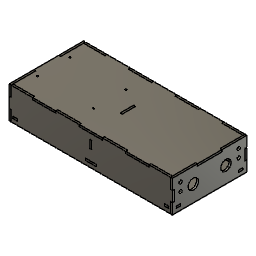
cessna-knobox-enclosure-v77 (Autodesk Fusion 360 design; units mm, degrees)
Autodesk Fusion 360 part; units mm, degrees
sketch "Sketch1" plane through (0, 0, 0) normal (0, 1, 0) x (1, 0, 0)
  line L0 (-146.75, 65) -> (146.75, 65)
  line L1 (146.75, 65) -> (146.75, -65)
  line L2 (146.75, -65) -> (-146.75, -65)
  line L3 (-146.75, -65) -> (-146.75, 65)
  line L4 (-136.75, -30) -> (-33.75, -30) construction
  circle A0 centre (-136.75, -30) radius 1.5
  circle A1 centre (-33.75, -30) radius 1.5
  line L5 (0, 0) -> (0, 38.2702) construction
  line L6 (-150.25, 68.5) -> (150.25, 68.5)
  line L7 (150.25, 68.5) -> (150.25, -68.5)
  line L8 (150.25, -68.5) -> (-150.25, -68.5)
  line L9 (-150.25, -68.5) -> (-150.25, 68.5)
  line L10 (-26.25, -24.7344) -> (-26.25, -4.7344) construction
  line L11 (-136.75, 30) -> (-33.75, 30) construction
  circle A2 centre (-136.75, 30) radius 1.5
  circle A3 centre (-33.75, 30) radius 1.5
  line L12 (-136.75, -30) -> (-136.75, -65) construction
  line L13 (-136.75, 30) -> (-136.75, -30) construction
  line L14 (-136.75, 30) -> (-136.75, 65) construction
  line L15 (0, 0) -> (35, 0) construction
  dimension "d1" = 103
  dimension "d2" = 3
  dimension "d3" = 3
  dimension "d4" = 130
  dimension "d5" = 10
  dimension "d7" = 3.5
  dimension "d9" = 3.5
  dimension "d10" = 3.5
  dimension "d11" = 3.5
  dimension "d20" = 7.5
  dimension "d21" = 173
  dimension "d36" = 103
  dimension "d37" = 3
  dimension "d38" = 3
  dimension "d39" = 60
  constraint horizontal L0
  constraint vertical L1
  constraint horizontal L2
  constraint vertical L3
  constraint horizontal L4
  constraint coincident L4.start A0.centre
  constraint coincident L4.end A1.centre
  constraint coincident L5.start L15.start
  constraint symmetric L0.start L0.end L5
  constraint horizontal L6
  constraint vertical L7
  constraint horizontal L8
  constraint vertical L9
  constraint horizontal L11
  constraint coincident L11.start A2.centre
  constraint coincident L11.end A3.centre
  constraint coincident L2 L12.end
  constraint perpendicular L2 L12
  constraint parallel L12 L13
  constraint coincident L0 L14.end
  constraint perpendicular L0 L14
  constraint equal L12 L14
  constraint perpendicular L5 L15
  constraint symmetric L0.start L2.end L15
  measures "d1" distance of L4.start L4.end
  measures "d2" diameter of A0
  measures "d3" diameter of A1
  measures "d4" distance of L0.start L2.end
  measures "d5" distance of L3 L4.start
  measures "d7" distance of L3 L9
  measures "d9" distance of L0 L6
  measures "d10" distance of L1 L7
  measures "d11" distance of L2 L8
  measures "d20" distance of L4.end L10
  measures "d21" distance of L1 L10
  measures "d36" distance of L11.end L11.start
  measures "d37" diameter of A2
  measures "d38" diameter of A3
  measures "d39" distance of L4 L11
extrude "Extrude1" add sketch "Sketch1" along normal blind 3.5 contours L0 L1 L2 L3 | L6 L7 L8 L9 makes body 1
extrude "Extrude2" add sketch "Sketch1" against normal blind 55 contours L6 L7 L8 L9 bodies 1
sketch "Sketch2" plane through (150.25, 0, 0) normal (1, 0, 0) x (0, 0, -1)
  line L0 (68.5, -55) -> (68.5, 3.5)
  line L1 (68.5, 3.5) -> (-68.5, 3.5)
  line L2 (-68.5, 3.5) -> (-68.5, -55)
  line L3 (-68.5, -55) -> (68.5, -55)
  line L4 (0, 3.5) -> (0, -55) construction
  circle A0 centre (30, -25.025) radius 9.5
  line L5 (68.5, 0) -> (-68.5, 0) construction
  line L6 (30, 0) -> (30, -55) construction
  line L7 (-30, 0) -> (-30, -55) construction
  circle A1 centre (-30, -25.025) radius 9.5
  line L8 (-30, -25.025) -> (30, -25.025) construction
  circle A2 centre (-53.5, -10.025) radius 3
  line L9 (-53.5, 3.5) -> (-53.5, -55) construction
  circle A3 centre (-53.5, -25.025) radius 3
  circle A4 centre (53.5, -10.025) radius 3
  circle A5 centre (53.5, -25.025) radius 3
  line L10 (53.5, 3.5) -> (53.5, -55) construction
  line L11 (-53.5, -10.025) -> (53.5, -10.025) construction
  line L12 (-53.5, -25.025) -> (53.5, -25.025) construction
  point P0 (-30, 0)
  point P1 (30, 0)
  dimension "d16" = 19
  dimension "d17" = 25.025
  dimension "d40" = 19
  dimension "d41" = 6
  dimension "d42" = 15
  dimension "d43" = 6
  dimension "d45" = 6
  dimension "d46" = 6
  dimension "d77" = 15
  constraint midpoint L1 L4.start
  constraint midpoint L3 L4.end
  constraint coincident P1 L6.start
  constraint coincident L3 L6.end
  constraint perpendicular L3 L6
  constraint coincident P0 L7.start
  constraint coincident L3 L7.end
  constraint perpendicular L3 L7
  constraint coincident A0.centre L6
  constraint coincident L7 A1.centre
  constraint coincident A1.centre L8.start
  constraint coincident A0.centre L8.end
  constraint parallel L3 L8
  constraint coincident L1 L9.start
  constraint coincident L3 L9.end
  constraint perpendicular L3 L9
  constraint coincident A2.centre L9
  constraint coincident L9 A3.centre
  constraint coincident L1 L10.start
  constraint coincident L3 L10.end
  constraint perpendicular L3 L10
  constraint symmetric L4 L9.start L10.start
  constraint coincident A4.centre L10
  constraint coincident A5.centre L10
  constraint coincident A2.centre L11.start
  constraint coincident A4.centre L11.end
  constraint coincident A3.centre L12.start
  constraint coincident A5.centre L12.end
  constraint parallel L8 L12
  constraint parallel L8 L11
  constraint coincident A1.centre L12
  measures "d16" diameter of A0
  measures "d17" distance of A0.centre L5
  measures "d40" diameter of A1
  measures "d41" diameter of A2
  measures "d42" distance of L2 L9
  measures "d43" diameter of A3
  measures "d45" diameter of A4
  measures "d46" diameter of A5
  measures "d77" distance of L11 L12
extrude "Extrude3" cut sketch "Sketch2" against normal blind 3.5 contours A0 | A1 | A2 | A3 | A4 | A5 bodies 1
sketch "Sketch3" plane through (0, 0, 68.5) normal (0, 0, 1) x (1, 0, 0)
  line L0 (150.25, -55) -> (150.25, 3.5)
  line L1 (150.25, 3.5) -> (-150.25, 3.5)
  line L2 (-150.25, 3.5) -> (-150.25, -55)
  line L3 (-150.25, -55) -> (150.25, -55)
  line L4 (150.25, 0) -> (-150.25, 0) construction
  line L5 (-150.25, -51.5) -> (150.25, -51.5) construction
  line L6 (-146.75, 3.5) -> (-146.75, -55) construction
  line L7 (146.75, 3.5) -> (146.75, -55) construction
  line L8 (0, 3.5) -> (0, -55) construction
  line L9 (-107.3214, 3.5) -> (-107.3214, -55) construction
  line L10 (-64.3929, 3.5) -> (-64.3929, -55) construction
  line L11 (-21.4643, 3.5) -> (-21.4643, -55) construction
  line L12 (21.4643, 3.5) -> (21.4643, -55) construction
  line L13 (64.3929, 3.5) -> (64.3929, -55) construction
  line L14 (107.3214, 3.5) -> (107.3214, -55) construction
  line L15 (-150.25, -25.75) -> (-107.3214, -25.75) construction
  line L16 (-107.3214, -25.75) -> (-64.3929, -25.75) construction
  line L17 (-64.3929, -25.75) -> (-21.4643, -25.75) construction
  line L18 (-21.4643, -25.75) -> (21.4643, -25.75) construction
  line L19 (21.4643, -25.75) -> (64.3929, -25.75) construction
  line L20 (64.3929, -25.75) -> (107.3214, -25.75) construction
  line L21 (107.3214, -25.75) -> (150.25, -25.75) construction
  line L22 (-150.25, -16) -> (150.25, -16) construction
  line L23 (-150.25, -35.5) -> (150.25, -35.5) construction
  line L24 (-127.3214, 3.5) -> (-127.3214, -16) construction
  line L25 (-127.3214, -16) -> (-127.3214, -35.5) construction
  line L26 (-127.3214, -35.5) -> (-127.3214, -55) construction
  line L27 (-150.25, -16) -> (-146.75, -16)
  line L28 (-146.75, -16) -> (-146.75, 3.5)
  line L29 (-107.3214, 3.5) -> (-107.3214, 0)
  line L30 (-107.3214, 0) -> (-64.3929, 0)
  line L31 (-64.3929, 0) -> (-64.3929, 3.5)
  line L32 (-21.4643, 3.5) -> (-21.4643, 0)
  line L33 (-21.4643, 0) -> (21.4643, 0)
  line L34 (21.4643, 0) -> (21.4643, 3.5)
  line L35 (64.3929, 3.5) -> (64.3929, 0)
  line L36 (64.3929, 0) -> (107.3214, 0)
  line L37 (107.3214, 0) -> (107.3214, 3.5)
  line L38 (146.75, 3.5) -> (146.75, -16)
  line L39 (146.75, -16) -> (150.25, -16)
  line L40 (-150.25, -35.5) -> (-146.75, -35.5)
  line L41 (-146.75, -35.5) -> (-146.75, -55)
  line L42 (150.25, -35.5) -> (146.75, -35.5)
  line L43 (146.75, -35.5) -> (146.75, -55)
  dimension "d22" = 3.5
  dimension "d23" = 3.5
  dimension "d24" = 3.5
  dimension "d25" = 20
  constraint coincident L2 L5.start
  constraint coincident L0 L5.end
  constraint perpendicular L0 L5
  constraint coincident L1 L6.start
  constraint coincident L3 L6.end
  constraint perpendicular L3 L6
  constraint coincident L1 L7.start
  constraint coincident L3 L7.end
  constraint perpendicular L3 L7
  constraint midpoint L1 L8.start
  constraint midpoint L3 L8.end
  constraint coincident L1 L9.start
  constraint coincident L3 L9.end
  constraint perpendicular L3 L9
  constraint coincident L1 L10.start
  constraint coincident L3 L10.end
  constraint perpendicular L5 L10
  constraint coincident L1 L11.start
  constraint coincident L3 L11.end
  constraint perpendicular L3 L11
  constraint coincident L1 L12.start
  constraint coincident L3 L12.end
  constraint perpendicular L3 L12
  constraint coincident L1 L13.start
  constraint coincident L3 L13.end
  constraint perpendicular L3 L13
  constraint coincident L1 L14.start
  constraint coincident L3 L14.end
  constraint perpendicular L3 L14
  constraint midpoint L2 L15.start
  constraint midpoint L9 L15.end
  constraint midpoint L10 L16.end
  constraint midpoint L11 L17.end
  constraint midpoint L12 L18.end
  constraint midpoint L13 L19.end
  constraint midpoint L14 L20.end
  constraint midpoint L0 L21.end
  constraint equal L15 L16
  constraint equal L16 L17
  constraint equal L17 L18
  constraint equal L18 L19
  constraint equal L19 L20
  constraint equal L20 L21
  constraint coincident L2 L22.start
  constraint coincident L0 L22.end
  constraint perpendicular L0 L22
  constraint coincident L2 L23.start
  constraint coincident L0 L23.end
  constraint perpendicular L0 L23
  constraint coincident L1 L24.start
  constraint coincident L22 L24.end
  constraint perpendicular L22 L24
  constraint coincident L23 L25.end
  constraint perpendicular L23 L25
  constraint coincident L3 L26.end
  constraint perpendicular L3 L26
  constraint equal L25 L26
  constraint equal L24 L25
  constraint coincident L6 L27.end
  constraint coincident L22 L27.end
  constraint coincident L4 L29.end
  constraint coincident L9 L29.end
  constraint coincident L4 L30.end
  constraint coincident L10 L30.end
  constraint coincident L4 L32.end
  constraint coincident L11 L32.end
  constraint coincident L4 L33.end
  constraint coincident L12 L33.end
  constraint coincident L4 L35.end
  constraint coincident L13 L35.end
  constraint coincident L4 L36.end
  constraint coincident L14 L36.end
  constraint coincident L7 L38.end
  constraint coincident L22 L38.end
  constraint coincident L6 L40.end
  constraint coincident L23 L40.end
  constraint coincident L7 L42.end
  constraint coincident L23 L42.end
  measures "d22" distance of L3 L5
  measures "d23" distance of L2 L6
  measures "d24" distance of L0 L7
  measures "d25" distance of L9 L24
sketch "Sketch4" plane through (0, 0, -68.5) normal (0, 0, -1) x (-1, 0, 0)
  line L0 (150.25, -55) -> (150.25, 3.5)
  line L1 (150.25, 3.5) -> (-150.25, 3.5)
  line L2 (-150.25, 3.5) -> (-150.25, -55)
  line L3 (-150.25, -55) -> (150.25, -55)
  line L4 (146.75, 3.5) -> (146.75, -55) construction
  line L5 (107.3214, 3.5) -> (107.3214, -55) construction
  line L6 (64.3929, 3.5) -> (64.3929, -55) construction
  line L7 (21.4643, 3.5) -> (21.4643, -55) construction
  line L8 (-21.4643, 3.5) -> (-21.4643, -55) construction
  line L9 (-64.3929, 3.5) -> (-64.3929, -55) construction
  line L10 (-107.3214, 3.5) -> (-107.3214, -55) construction
  line L11 (150.25, -16) -> (-150.25, -16) construction
  line L12 (150.25, -35.5) -> (-150.25, -35.5) construction
  line L13 (-146.75, 3.5) -> (-146.75, -55) construction
  line L14 (-150.25, -16) -> (-146.75, -16)
  line L15 (-146.75, -16) -> (-146.75, 3.5)
  line L16 (-150.25, 0) -> (150.25, 0) construction
  line L17 (-107.3214, 3.5) -> (-107.3214, 0)
  line L18 (-107.3214, 0) -> (-64.3929, 0)
  line L19 (-64.3929, 0) -> (-64.3929, 3.5)
  line L20 (-21.4643, 3.5) -> (-21.4643, 0)
  line L21 (-21.4643, 0) -> (21.4643, 0)
  line L22 (21.4643, 0) -> (21.4643, 3.5)
  line L23 (64.3929, 3.5) -> (64.3929, 0)
  line L24 (64.3929, 0) -> (107.3214, 0)
  line L25 (107.3214, 0) -> (107.3214, 3.5)
  line L26 (146.75, 3.5) -> (146.75, -16)
  line L27 (146.75, -16) -> (150.25, -16)
  line L28 (150.25, -35.5) -> (146.75, -35.5)
  line L29 (146.75, -35.5) -> (146.75, -55)
  line L30 (-150.25, -35.5) -> (-146.75, -35.5)
  line L31 (-146.75, -35.5) -> (-146.75, -55)
  constraint coincident L11.end L14.start
  constraint coincident L13 L14.end
  constraint coincident L11 L14.end
  constraint coincident L13.start L15.end
  constraint coincident L10.start L17.start
  constraint coincident L10 L17.end
  constraint coincident L16 L17.end
  constraint coincident L9 L18.end
  constraint coincident L16 L18.end
  constraint coincident L9.start L19.end
  constraint coincident L8.start L20.start
  constraint coincident L8 L20.end
  constraint coincident L16 L20.end
  constraint coincident L7 L21.end
  constraint coincident L16 L21.end
  constraint coincident L7.start L22.end
  constraint coincident L6.start L23.start
  constraint coincident L6 L23.end
  constraint coincident L16 L23.end
  constraint coincident L5 L24.end
  constraint coincident L16 L24.end
  constraint coincident L5.start L25.end
  constraint coincident L4.start L26.start
  constraint coincident L4 L26.end
  constraint coincident L11 L26.end
  constraint coincident L11.start L27.end
  constraint coincident L12.start L28.start
  constraint coincident L4 L28.end
  constraint coincident L12 L28.end
  constraint coincident L4.end L29.end
  constraint coincident L12.end L30.start
  constraint coincident L12 L30.end
  constraint coincident L13 L30.end
  constraint coincident L13.end L31.end
extrude "Extrude4" add sketch "Sketch3" against normal blind 3.5 separate body contours L0 L1 L2 L3 L27 L28 L29 L30 L31 L32 L33 L34 L35 L36 L37 L38 L39 L40 L41 L42 L43 makes body 2
extrude "Extrude5" add sketch "Sketch4" against normal blind 3.5 separate body contours L0 L1 L2 L3 L14 L15 L17 L18 L19 L20 L21 L22 L23 L24 L25 L26 L27 L28 L29 L30 L31 makes body 3
combine "Combine1" operation cut target body 1 tool bodies 2 3 keep tools
sketch "Sketch5" plane through (150.25, 0, 0) normal (1, 0, 0) x (0, 0, -1)
  circle A0 centre (30, -25.025) radius 9.5
  line L0 (68.5, -35.5) -> (65, -35.5)
  line L1 (65, -35.5) -> (65, -16)
  line L2 (65, -16) -> (68.5, -16)
  line L3 (68.5, -16) -> (68.5, 3.5)
  line L4 (68.5, 3.5) -> (-68.5, 3.5)
  line L5 (-68.5, 3.5) -> (-68.5, -16)
  line L6 (-68.5, -16) -> (-65, -16)
  line L7 (-65, -16) -> (-65, -35.5)
  line L8 (-65, -35.5) -> (-68.5, -35.5)
  line L9 (-68.5, -35.5) -> (-68.5, -55)
  line L10 (-68.5, -55) -> (68.5, -55)
  line L11 (68.5, -55) -> (68.5, -35.5)
  line L12 (0, 3.5) -> (0, -55) construction
  line L13 (-22.8333, 3.5) -> (-22.8333, -55) construction
  line L14 (22.8333, 3.5) -> (22.8333, -55) construction
  line L15 (-68.5, -45.25) -> (-22.8333, -45.25) construction
  line L16 (-22.8333, -45.25) -> (22.8333, -45.25) construction
  line L17 (22.8333, -45.25) -> (68.5, -45.25) construction
  line L18 (-68.5, 0) -> (68.5, 0) construction
  line L19 (-22.8333, 3.5) -> (-22.8333, 0)
  line L20 (-22.8333, 0) -> (22.8333, 0)
  line L21 (22.8333, 0) -> (22.8333, 3.5)
  circle A1 centre (-30, -25.025) radius 9.5
  circle A2 centre (-53.5, -25.025) radius 3
  circle A3 centre (53.5, -10.025) radius 3
  circle A4 centre (-53.5, -10.025) radius 3
  circle A5 centre (53.5, -25.025) radius 3
  dimension "d31" = 3.5
  constraint midpoint L4 L12.start
  constraint midpoint L10 L12.end
  constraint coincident L4 L13.start
  constraint coincident L10 L13.end
  constraint perpendicular L10 L13
  constraint coincident L4 L14.start
  constraint coincident L10 L14.end
  constraint perpendicular L10 L14
  constraint symmetric L12 L13 L14
  constraint midpoint L9 L15.start
  constraint coincident L13 L15.end
  constraint perpendicular L13 L15
  constraint coincident L14 L16.end
  constraint perpendicular L14 L16
  constraint midpoint L11 L17.end
  constraint perpendicular L11 L17
  constraint equal L16 L17
  constraint coincident L5 L18.start
  constraint coincident L3 L18.end
  constraint perpendicular L3 L18
  constraint coincident L18 L19.end
  constraint coincident L13 L19.end
  constraint coincident L18 L20.end
  constraint coincident L14 L20.end
  measures "d31" distance of L4 L18
extrude "Extrude6" add sketch "Sketch5" against normal blind 3.5 separate body contours L0 L1 L2 L3 L4 L5 L6 L7 L8 L9 L10 L11 L19 L20 L21 makes body 4
sketch "Sketch6" plane through (-150.25, 0, 0) normal (-1, 0, 0) x (0, 0, 1)
  line L0 (-68.5, -16) -> (-65, -16)
  line L1 (-65, -16) -> (-65, -35.5)
  line L2 (-65, -35.5) -> (-68.5, -35.5)
  line L3 (-68.5, -35.5) -> (-68.5, -55)
  line L4 (-68.5, -55) -> (68.5, -55)
  line L5 (68.5, -55) -> (68.5, -35.5)
  line L6 (68.5, -35.5) -> (65, -35.5)
  line L7 (65, -35.5) -> (65, -16)
  line L8 (65, -16) -> (68.5, -16)
  line L9 (68.5, -16) -> (68.5, 3.5)
  line L10 (68.5, 3.5) -> (-68.5, 3.5)
  line L11 (-68.5, 3.5) -> (-68.5, -16)
  line L12 (-22.8333, 0) -> (-22.8333, 3.5)
  line L13 (22.8333, 0) -> (-22.8333, 0)
  line L14 (22.8333, 3.5) -> (22.8333, 0)
extrude "Extrude7" add sketch "Sketch6" against normal blind 3.5 separate body contours L0 L1 L2 L3 L4 L5 L6 L7 L8 L9 L10 L11 L12 L13 L14 makes body 5
combine "Combine2" operation cut target body 1 tool bodies 4 5 keep tools
sketch "Sketch7" plane through (-150.25, 0, 0) normal (-1, 0, 0) x (0, 0, 1)
  line L0 (22.8333, 3.5) -> (22.8333, 0)
  line L1 (22.8333, 0) -> (-22.8333, 0)
  line L2 (-22.8333, 0) -> (-22.8333, 3.5)
  line L3 (-22.8333, 3.5) -> (-68.5, 3.5)
  line L4 (-68.5, 3.5) -> (-68.5, -16)
  line L5 (-68.5, -16) -> (-65, -16)
  line L6 (-65, -16) -> (-65, -35.5)
  line L7 (-65, -35.5) -> (-68.5, -35.5)
  line L8 (-68.5, -35.5) -> (-68.5, -55)
  line L9 (-68.5, -55) -> (68.5, -55)
  line L10 (68.5, -55) -> (68.5, -35.5)
  line L11 (68.5, -35.5) -> (65, -35.5)
  line L12 (65, -35.5) -> (65, -16)
  line L13 (65, -16) -> (68.5, -16)
  line L14 (68.5, -16) -> (68.5, 3.5)
  line L15 (68.5, 3.5) -> (22.8333, 3.5)
sketch "Sketch12" plane through (-150.25, -23.25, 0) normal (-1, 0, 0) x (0, 0, 1)
  line L0 (0, 23.25) -> (0, -25) construction
  circle A0 centre (-15, 8.25) radius 1.5
  circle A1 centre (15, 8.25) radius 1.5
  line L1 (-15, 8.25) -> (15, 8.25) construction
  line L2 (68.5, 23.25) -> (-68.5, 23.25) construction
  circle A2 centre (-30, -1.775) radius 9.5 construction
  circle A3 centre (30, -1.775) radius 9.5 construction
  line L3 (-30, -1.775) -> (-30, -27) construction
  line L4 (-68.5, -31.75) -> (68.5, -31.75) construction
  line L5 (-6.02, 13.7) -> (6.02, 13.7)
  line L6 (6.02, 13.7) -> (6.02, 2.8)
  line L7 (6.02, 2.8) -> (-6.02, 2.8)
  line L8 (-6.02, 2.8) -> (-6.02, 13.7)
  point P0 (0, 23.25)
  dimension "d47" = 3
  dimension "d48" = 3
  dimension "d49" = 30
  dimension "d52" = 10.9
  dimension "d53" = 12.04
  dimension "d56" = 15
  constraint coincident P0 L0.start
  constraint vertical L0
  constraint coincident A0.centre L1.start
  constraint coincident A1.centre L1.end
  constraint perpendicular L0 L1
  constraint symmetric L0 A0.centre A1.centre
  constraint coincident A2.centre L3.start
  constraint perpendicular L1 L3
  constraint horizontal L5
  constraint vertical L6
  constraint horizontal L7
  constraint vertical L8
  constraint symmetric L0 L6.end L7.end
  constraint symmetric L1 L5.start L7.end
  measures "d47" diameter of A0
  measures "d48" diameter of A1
  measures "d49" distance of A0.centre A1.centre
  measures "d52" distance of L5.start L7.end
  measures "d53" distance of L5.start L5.end
  measures "d56" distance of L1 L2
extrude "Extrude8" cut sketch "Sketch12" against normal blind 3.5 bodies 5
ref_plane "WorkPlane1" through (-148.5, -51.5, 0) normal (0, -1, 0) x (0, 0, -1)
sketch "Sketch13" plane through (-148.5, -51.5, 0) normal (0, -1, 0) x (1, 0, 0)
  line L0 (1.75, 68.5) -> (1.75, -68.5)
  line L1 (1.75, -65) -> (295.25, -65)
  line L2 (1.75, -65) -> (1.75, -50)
  arc A0 (16.75, -65) -> (1.75, -50) centre (1.75, -65) ccw
  line L3 (1.75, -65) -> (16.75, -65)
  dimension "d58" = 15
  constraint coincident L1.start L2.start
  constraint perpendicular L1 L2
  measures "d58" distance of L1.start L2.end
extrude "Extrude9" add sketch "Sketch13" against normal blind 10.5 separate body makes body 6
ref_plane "WorkPlane2" through (-139.25, -48, -57.5) normal (0, -1, 0) x (1, 0, 0)
ref_plane "WorkPlane3" through (-139.25, -44.5, -57.5) normal (0, -1, 0) x (1, 0, 0)
split "Split1" by plane through (-139.25, -44.5, -57.5) normal (0, -1, 0) and through (-139.25, -48, -57.5) normal (0, -1, 0) bodies 6 makes body 7 at (-143.9112, -45.6667, -50.2711) makes body 8 at (-144.6298, -51.5, -55.2534)
sketch "Sketch14" plane through (0, 0, -65) normal (0, 0, -1) x (-1, 0, 0)
  line L0 (131.75, -48) -> (146.75, -48)
  line L1 (146.75, -48) -> (146.75, -44.5)
  line L2 (146.75, -44.5) -> (131.75, -44.5)
  line L3 (131.75, -44.5) -> (131.75, -48)
  line L4 (139.25, -44.5) -> (139.25, -48) construction
  line L5 (135.25, -44.5) -> (135.25, -48)
  line L6 (143.25, -44.5) -> (143.25, -48)
  dimension "d63" = 8
  constraint midpoint L2 L4.start
  constraint midpoint L0 L4.end
  constraint coincident L2 L5.start
  constraint coincident L0 L5.end
  constraint perpendicular L0 L5
  constraint coincident L2 L6.start
  constraint coincident L0 L6.end
  constraint perpendicular L0 L6
  constraint symmetric L4 L5.start L6.start
  measures "d63" distance of L5 L6
extrude "Extrude10" add sketch "Sketch14" along normal blind 3.5 contours L0 L2 L5 L6 bodies 7
sketch "Sketch15" plane through (-146.75, 0, 0) normal (-1, 0, 0) x (0, 0, 1)
  line L0 (-65, -48) -> (-50, -48)
  line L1 (-50, -48) -> (-50, -44.5)
  line L2 (-50, -44.5) -> (-65, -44.5)
  line L3 (-65, -44.5) -> (-65, -48)
  line L4 (-57.5, -44.5) -> (-57.5, -48) construction
  line L5 (-61.5, -44.5) -> (-61.5, -48)
  line L6 (-53.5, -44.5) -> (-53.5, -48)
  dimension "d66" = 8
  constraint midpoint L2 L4.start
  constraint midpoint L0 L4.end
  constraint coincident L2 L5.start
  constraint coincident L0 L5.end
  constraint perpendicular L0 L5
  constraint coincident L2 L6.start
  constraint coincident L0 L6.end
  constraint perpendicular L0 L6
  constraint symmetric L4 L5.start L6.start
  measures "d66" distance of L5 L6
extrude "Extrude11" add sketch "Sketch15" along normal blind 3.5 contours L0 L2 L5 L6 bodies 7
sketch "Sketch16" plane through (0, -48, 0) normal (0, -1, 0) x (1, 0, 0)
  line L0 (-146.75, -65) -> (-143.25, -65)
  line L1 (-143.25, -65) -> (-143.25, -68.5)
  line L2 (-143.25, -68.5) -> (-135.25, -68.5)
  line L3 (-135.25, -68.5) -> (-135.25, -65)
  line L4 (-135.25, -65) -> (-131.75, -65)
  arc A0 (-131.75, -65) -> (-146.75, -50) centre (-146.75, -65) ccw
  line L5 (-146.75, -50) -> (-146.75, -53.5)
  line L6 (-146.75, -53.5) -> (-150.25, -53.5)
  line L7 (-150.25, -53.5) -> (-150.25, -61.5)
  line L8 (-150.25, -61.5) -> (-146.75, -61.5)
  line L9 (-146.75, -61.5) -> (-146.75, -65)
  line L10 (-142.5, -55.9689) -> (-144.25, -59)
  line L11 (-144.25, -59) -> (-142.5, -62.0311)
  line L12 (-142.5, -62.0311) -> (-139, -62.0311)
  line L13 (-139, -62.0311) -> (-137.25, -59)
  line L14 (-137.25, -59) -> (-139, -55.9689)
  line L15 (-139, -55.9689) -> (-142.5, -55.9689)
  line L16 (-150.25, -59) -> (-133.0023, -59) construction
  line L17 (-140.75, -68.5) -> (-140.75, -51.2523) construction
  point P0 (-140.75, -59)
  dimension "d69" = 3.5
  dimension "d70" = 2.5
  dimension "d71" = 2.5
  constraint coincident L7 L16.start
  constraint coincident A0 L16.end
  constraint perpendicular L7 L16
  constraint coincident L2 L17.start
  constraint coincident A0 L17.end
  constraint perpendicular L16 L17
  constraint coincident P0 L16
  constraint coincident P0 L17
  constraint parallel L15 L16
  measures "d69" distance of L10.start P0
  measures "d70" distance of L8 L16
  measures "d71" distance of L1 L17
extrude "Extrude12" cut sketch "Sketch16" against normal blind 3.5 contours L10 L11 L12 L13 L14 L15 bodies 7
sketch "Sketch17" plane through (0, -51.5, 0) normal (0, -1, 0) x (1, 0, 0)
  line L0 (-146.75, -65) -> (-131.75, -65)
  arc A0 (-131.75, -65) -> (-146.75, -50) centre (-146.75, -65) ccw
  line L1 (-146.75, -50) -> (-146.75, -65)
  line L2 (-139, -55.9689) -> (-142.5, -55.9689) construction
  line L3 (-142.5, -55.9689) -> (-144.25, -59) construction
  line L4 (-144.25, -59) -> (-142.5, -62.0311) construction
  line L5 (-142.5, -62.0311) -> (-139, -62.0311) construction
  line L6 (-139, -62.0311) -> (-137.25, -59) construction
  line L7 (-137.25, -59) -> (-139, -55.9689) construction
  circle A1 centre (-140.75, -59) radius 1.5
  point P0 (-140.75, -59)
  dimension "d74" = 3
  constraint coincident P0 A1.centre
  measures "d74" diameter of A1
extrude "Extrude13" cut sketch "Sketch17" against normal blind 10.5 contours A1 bodies 6 8
copy_body "CopyPasteBodies1" bodies 7 8 6 makes body 9 makes body 10 makes body 11
move_body "Move1" bodies 9 10 11 to x (0, 0, 1) y (0, 1, 0) z (-1, 0, 0) at (81.75, 0, 81.75)
copy_body "CopyPasteBodies2" bodies 9 10 11 makes body 12 makes body 13 makes body 14
move_body "Move2" bodies 12 13 14 to x (0, 0, 1) y (0, 1, 0) z (-1, 0, 0) at (81.75, 0, -81.75)
copy_body "CopyPasteBodies3" bodies 6 7 8 makes body 15 makes body 16 makes body 17
move_body "Move3" bodies 15 16 17 to x (0, 0, -1) y (0, 1, 0) z (1, 0, 0) at (-81.75, 0, -81.75)
combine "Combine3" operation cut target body 2 tool bodies 16 12 keep tools
combine "Combine4" operation cut target body 3 tool bodies 7 9 keep tools
combine "Combine5" operation cut target body 5 tool bodies 16 7 keep tools
combine "Combine6" operation cut target body 4 tool bodies 12 9 keep tools
ref_plane "WorkPlane4" through (-1.75, -25.75, 0) normal (1, 0, 0) x (0, 0, -1)
sketch "Sketch19" plane through (-1.75, -25.75, 0) normal (1, 0, 0) x (0, 0, -1)
  line L0 (-65, 9.75) -> (-65, -9.75)
  line L1 (65, -9.75) -> (65, 9.75)
  line L2 (-22.8333, 25.75) -> (22.8333, 25.75)
  line L3 (-65, -9.75) -> (-65, 25.75)
  line L4 (-65, 25.75) -> (65, 25.75)
  line L5 (65, 25.75) -> (65, -9.75)
  line L6 (-65, -9.75) -> (-61, -9.75)
  line L7 (-61, -9.75) -> (-61, 21.75)
  line L8 (-61, 21.75) -> (61, 21.75)
  line L9 (65, -9.75) -> (61, -9.75)
  line L10 (61, -9.75) -> (61, 21.75)
  dimension "d81" = 4
  dimension "d82" = 4
  dimension "d83" = 4
  constraint coincident L0.end L3.start
  constraint perpendicular L2 L3
  constraint perpendicular L1 L4
  constraint coincident L1.start L5.end
  constraint perpendicular L4 L5
  constraint coincident L2.end L4
  constraint perpendicular L3 L6
  constraint perpendicular L4 L7
  constraint perpendicular L5 L8
  constraint perpendicular L1 L9
  constraint perpendicular L4 L10
  measures "d81" distance of L0.end L6.end
  measures "d82" distance of L4 L8
  measures "d83" distance of L1.start L9.end
extrude "Extrude16" add sketch "Sketch19" along normal blind 3.5 separate body makes body 18
sketch "Sketch20" plane through (0, 0, -65) normal (0, 0, -1) x (-1, 0, 0)
  line L0 (1.75, -35.5) -> (1.75, 0)
  line L1 (1.75, 0) -> (-1.75, 0)
  line L2 (-1.75, 0) -> (-1.75, -35.5)
  line L3 (-1.75, -35.5) -> (1.75, -35.5)
  line L4 (-1.75, -17.75) -> (1.75, -17.75) construction
  line L5 (-1.75, -10.25) -> (1.75, -10.25)
  line L6 (-1.75, -25.25) -> (1.75, -25.25)
  dimension "d88" = 15
  constraint midpoint L2 L4.start
  constraint midpoint L0 L4.end
  constraint coincident L2 L5.start
  constraint coincident L0 L5.end
  constraint perpendicular L0 L5
  constraint coincident L2 L6.start
  constraint coincident L0 L6.end
  constraint perpendicular L0 L6
  constraint symmetric L4 L5.start L6.start
  measures "d88" distance of L5 L6
extrude "Extrude17" add sketch "Sketch20" along normal blind 3.5 contours L0 L2 L5 L6 bodies 18
sketch "Sketch21" plane through (0, 0, 65) normal (0, 0, 1) x (1, 0, 0)
  line L0 (-1.75, 0) -> (-1.75, -35.5)
  line L1 (-1.75, -35.5) -> (1.75, -35.5)
  line L2 (1.75, -35.5) -> (1.75, 0)
  line L3 (1.75, 0) -> (-1.75, 0)
  line L4 (1.75, -10.25) -> (-1.75, -10.25)
  line L5 (1.75, -25.25) -> (-1.75, -25.25)
extrude "Extrude18" add sketch "Sketch21" along normal blind 3.5 contours L0 L2 L4 L5 bodies 18
sketch "Sketch22" plane through (0, 0, 0) normal (0, 1, 0) x (-1, 0, 0)
  line L0 (1.75, -65) -> (1.75, 65)
  line L1 (1.75, 65) -> (-1.75, 65)
  line L2 (-1.75, 65) -> (-1.75, -65)
  line L3 (-1.75, -65) -> (1.75, -65)
  line L4 (1.75, 0) -> (-1.75, 0) construction
  line L5 (1.75, -12.5) -> (-1.75, -12.5)
  line L6 (1.75, 12.5) -> (-1.75, 12.5)
  dimension "d93" = 25
  constraint midpoint L0 L4.start
  constraint midpoint L2 L4.end
  constraint coincident L0 L5.start
  constraint coincident L2 L5.end
  constraint perpendicular L2 L5
  constraint coincident L0 L6.start
  constraint coincident L2 L6.end
  constraint perpendicular L2 L6
  constraint symmetric L4 L5.end L6.end
  measures "d93" distance of L5 L6
extrude "Extrude19" add sketch "Sketch22" along normal blind 3.5 contours L0 L2 L5 L6 bodies 18
combine "Combine7" operation cut target body 1 tool bodies 18 keep tools
combine "Combine8" operation cut target body 2 tool bodies 18 keep tools
combine "Combine9" operation cut target body 3 tool bodies 18 keep tools
sketch "bottom" plane through (0, 3.5, 0) normal (0, 1, 0) x (-1, 0, 0)
  line L0 (-1.75, 12.5) -> (1.75, 12.5)
  line L1 (1.75, 12.5) -> (1.75, -12.5)
  line L2 (1.75, -12.5) -> (-1.75, -12.5)
  line L3 (-1.75, -12.5) -> (-1.75, 12.5)
  line L4 (146.75, -22.8333) -> (150.25, -22.8333)
  line L5 (150.25, -22.8333) -> (150.25, 22.8333)
  line L6 (150.25, 22.8333) -> (146.75, 22.8333)
  line L7 (146.75, 22.8333) -> (146.75, 65)
  line L8 (146.75, 65) -> (107.3214, 65)
  line L9 (107.3214, 65) -> (107.3214, 68.5)
  line L10 (107.3214, 68.5) -> (64.3929, 68.5)
  line L11 (64.3929, 68.5) -> (64.3929, 65)
  line L12 (64.3929, 65) -> (21.4643, 65)
  line L13 (21.4643, 65) -> (21.4643, 68.5)
  line L14 (21.4643, 68.5) -> (-21.4643, 68.5)
  line L15 (-21.4643, 68.5) -> (-21.4643, 65)
  line L16 (-21.4643, 65) -> (-64.3929, 65)
  line L17 (-64.3929, 65) -> (-64.3929, 68.5)
  line L18 (-64.3929, 68.5) -> (-107.3214, 68.5)
  line L19 (-107.3214, 68.5) -> (-107.3214, 65)
  line L20 (-107.3214, 65) -> (-146.75, 65)
  line L21 (-146.75, 65) -> (-146.75, 22.8333)
  line L22 (-146.75, 22.8333) -> (-150.25, 22.8333)
  line L23 (-150.25, 22.8333) -> (-150.25, -22.8333)
  line L24 (-150.25, -22.8333) -> (-146.75, -22.8333)
  line L25 (-146.75, -22.8333) -> (-146.75, -65)
  line L26 (-146.75, -65) -> (-107.3214, -65)
  line L27 (-107.3214, -65) -> (-107.3214, -68.5)
  line L28 (-107.3214, -68.5) -> (-64.3929, -68.5)
  line L29 (-64.3929, -68.5) -> (-64.3929, -65)
  line L30 (-64.3929, -65) -> (-21.4643, -65)
  line L31 (-21.4643, -65) -> (-21.4643, -68.5)
  line L32 (-21.4643, -68.5) -> (21.4643, -68.5)
  line L33 (21.4643, -68.5) -> (21.4643, -65)
  line L34 (21.4643, -65) -> (64.3929, -65)
  line L35 (64.3929, -65) -> (64.3929, -68.5)
  line L36 (64.3929, -68.5) -> (107.3214, -68.5)
  line L37 (107.3214, -68.5) -> (107.3214, -65)
  line L38 (107.3214, -65) -> (146.75, -65)
  line L39 (146.75, -65) -> (146.75, -22.8333)
  circle A0 centre (136.75, 30) radius 1.5
  circle A1 centre (33.75, 30) radius 1.5
  circle A2 centre (136.75, -30) radius 1.5
  circle A3 centre (33.75, -30) radius 1.5
sketch "back" plane through (-150.25, 0, 0) normal (-1, 0, 0) x (0, 0, 1)
  line L0 (-61.5, -48) -> (-61.5, -44.5)
  line L1 (-61.5, -44.5) -> (-53.5, -44.5)
  line L2 (-53.5, -44.5) -> (-53.5, -48)
  line L3 (-53.5, -48) -> (-61.5, -48)
  line L4 (53.5, -48) -> (53.5, -44.5)
  line L5 (53.5, -44.5) -> (61.5, -44.5)
  line L6 (61.5, -44.5) -> (61.5, -48)
  line L7 (61.5, -48) -> (53.5, -48)
  line L8 (6.02, -9.55) -> (6.02, -20.45)
  line L9 (6.02, -20.45) -> (-6.02, -20.45)
  line L10 (-6.02, -20.45) -> (-6.02, -9.55)
  line L11 (-6.02, -9.55) -> (6.02, -9.55)
  circle A0 centre (-15, -15) radius 1.5
  circle A1 centre (15, -15) radius 1.5
  line L12 (22.8333, 3.5) -> (22.8333, 0)
  line L13 (22.8333, 0) -> (-22.8333, 0)
  line L14 (-22.8333, 0) -> (-22.8333, 3.5)
  line L15 (-22.8333, 3.5) -> (-68.5, 3.5)
  line L16 (-68.5, 3.5) -> (-68.5, -16)
  line L17 (-68.5, -16) -> (-65, -16)
  line L18 (-65, -16) -> (-65, -35.5)
  line L19 (-65, -35.5) -> (-68.5, -35.5)
  line L20 (-68.5, -35.5) -> (-68.5, -55)
  line L21 (-68.5, -55) -> (68.5, -55)
  line L22 (68.5, -55) -> (68.5, -35.5)
  line L23 (68.5, -35.5) -> (65, -35.5)
  line L24 (65, -35.5) -> (65, -16)
  line L25 (65, -16) -> (68.5, -16)
  line L26 (68.5, -16) -> (68.5, 3.5)
  line L27 (68.5, 3.5) -> (22.8333, 3.5)
sketch "front" plane through (150.25, 0, 0) normal (1, 0, 0) x (0, 0, -1)
  line L0 (53.5, -48) -> (53.5, -44.5)
  line L1 (53.5, -44.5) -> (61.5, -44.5)
  line L2 (61.5, -44.5) -> (61.5, -48)
  line L3 (61.5, -48) -> (53.5, -48)
  line L4 (-61.5, -48) -> (-61.5, -44.5)
  line L5 (-61.5, -44.5) -> (-53.5, -44.5)
  line L6 (-53.5, -44.5) -> (-53.5, -48)
  line L7 (-53.5, -48) -> (-61.5, -48)
  circle A0 centre (-30, -25.025) radius 9.5
  circle A1 centre (53.5, -10.025) radius 3
  circle A2 centre (-53.5, -10.025) radius 3
  circle A3 centre (-53.5, -25.025) radius 3
  circle A4 centre (53.5, -25.025) radius 3
  circle A5 centre (30, -25.025) radius 9.5
  line L8 (-22.8333, 3.5) -> (-68.5, 3.5)
  line L9 (-68.5, 3.5) -> (-68.5, -16)
  line L10 (-68.5, -16) -> (-65, -16)
  line L11 (-65, -16) -> (-65, -35.5)
  line L12 (-65, -35.5) -> (-68.5, -35.5)
  line L13 (-68.5, -35.5) -> (-68.5, -55)
  line L14 (-68.5, -55) -> (68.5, -55)
  line L15 (68.5, -55) -> (68.5, -35.5)
  line L16 (68.5, -35.5) -> (65, -35.5)
  line L17 (65, -35.5) -> (65, -16)
  line L18 (65, -16) -> (68.5, -16)
  line L19 (68.5, -16) -> (68.5, 3.5)
  line L20 (68.5, 3.5) -> (22.8333, 3.5)
  line L21 (22.8333, 3.5) -> (22.8333, 0)
  line L22 (22.8333, 0) -> (-22.8333, 0)
  line L23 (-22.8333, 0) -> (-22.8333, 3.5)
ref_plane "WorkPlane5" through (0, -51.5, 66.75) normal (0, -1, 0) x (-1, 0, 0)
sketch "Sketch33" plane through (0, -51.5, 66.75) normal (0, -1, 0) x (1, 0, 0)
  line L0 (0, -7.75) -> (0, 0) construction
  circle A0 centre (0, -7.75) radius 1.5
  arc A1 (-15, -1.75) -> (15, -1.75) centre (0, -1.75) ccw
  line L1 (146.75, -1.75) -> (-146.75, -1.75)
  dimension "d97" = 3
  dimension "d111" = 15
  dimension "d112" = 6
  constraint coincident L0.end origin
  constraint coincident L0.start A0.centre
  constraint symmetric L0 A1.start A1.end
  constraint coincident L0 A1.centre
  constraint coincident A1.start L1
  constraint coincident A1.end L1
  constraint coincident A1.centre L1
  measures "d97" diameter of A0
  measures "d111" radius of A1
  measures "d112" distance of L0.start L1
extrude "Extrude20" add sketch "Sketch33" against normal blind 3.5 separate body makes body 19
sketch "Sketch34" plane through (0, -48, 0) normal (0, 1, 0) x (-1, 0, 0)
  circle A0 centre (0, 59) radius 1.5
  line L0 (1.75, 55.9689) -> (3.5, 59)
  line L1 (3.5, 59) -> (1.75, 62.0311)
  line L2 (1.75, 62.0311) -> (-1.75, 62.0311)
  line L3 (-1.75, 62.0311) -> (-3.5, 59)
  line L4 (-3.5, 59) -> (-1.75, 55.9689)
  line L5 (-1.75, 55.9689) -> (1.75, 55.9689)
  arc A1 (-15, 65) -> (15, 65) centre (0, 65) ccw
  line L6 (15, 65) -> (-15, 65)
  line L7 (15, 65) -> (-15, 65)
  point P0 (0, 59)
  point P1 (0, 59)
  dimension "d101" = 3.5
  constraint coincident P1 P0
  constraint coincident A1.end L6.start
  constraint coincident A1.start L6.end
  constraint parallel L5 L6
  measures "d101" distance of L0.start P1
extrude "Extrude21" add sketch "Sketch34" along normal blind 3.5 separate body contours A1 L6 L7 makes body 20
sketch "Sketch35" plane through (0, -44.5, 0) normal (0, 1, 0) x (-1, 0, 0)
  circle A0 centre (0, 59) radius 1.5
  line L0 (1.75, 55.9689) -> (-1.75, 55.9689)
  line L1 (-1.75, 55.9689) -> (-3.5, 59)
  line L2 (-3.5, 59) -> (-1.75, 62.0311)
  line L3 (-1.75, 62.0311) -> (1.75, 62.0311)
  line L4 (1.75, 62.0311) -> (3.5, 59)
  line L5 (3.5, 59) -> (1.75, 55.9689)
  line L6 (15, 65) -> (-15, 65)
  arc A1 (-15, 65) -> (15, 65) centre (0, 65) ccw
  point P0 (0, 59)
  dimension "d104" = 3
  constraint coincident P0 A0.centre
  measures "d104" diameter of A0
extrude "Extrude22" add sketch "Sketch35" along normal blind 3.5 separate body contours L0 L1 L2 L3 L4 L5 | L6 A1 makes body 21
sketch "Sketch36" plane through (0, 0, 65) normal (0, 0, 1) x (1, 0, 0)
  line L0 (-15, -48) -> (15, -48)
  line L1 (15, -48) -> (15, -44.5)
  line L2 (15, -44.5) -> (-15, -44.5)
  line L3 (-15, -44.5) -> (-15, -48)
  line L4 (-10, -44.5) -> (-10, -48)
  line L5 (10, -44.5) -> (10, -48)
  line L6 (0, -48) -> (0, -44.5) construction
  dimension "d107" = 5
  constraint coincident L2 L4.start
  constraint coincident L0 L4.end
  constraint perpendicular L0 L4
  constraint coincident L2 L5.start
  constraint coincident L0 L5.end
  constraint perpendicular L0 L5
  constraint midpoint L0 L6.start
  constraint midpoint L2 L6.end
  constraint symmetric L4.start L5.start L6
  measures "d107" distance of L1 L5
extrude "Extrude23" add sketch "Sketch36" along normal blind 3.5 contours L0 L2 L4 L5 bodies 20
copy_body "CopyPasteBodies4" bodies 19 20 21 makes body 22 makes body 23 makes body 24
move_body "Move4" bodies 22 23 24 to x (-1, 0, 0) y (0, 1, 0) z (0, 0, -1) at (-1, 0, 0)
sketch "Sketch18" plane through (0, -51.5, 0) normal (0, -1, 0) x (1, 0, 0)
  circle A0 centre (-140.75, 59) radius 1.5
  line L0 (-146.75, 65) -> (-146.75, 50)
  arc A1 (-146.75, 50) -> (-131.75, 65) centre (-146.75, 65) ccw construction
  line L1 (-131.75, 65) -> (-146.75, 65)
  line L2 (-146.75, 65) -> (146.75, 65)
  line L3 (146.75, 65) -> (146.75, -65)
  line L4 (146.75, -65) -> (-146.75, -65)
  line L5 (-146.75, -65) -> (-146.75, 65)
  circle A2 centre (-140.75, -59) radius 1.5
  circle A3 centre (140.75, -59) radius 1.5
  circle A4 centre (140.75, 59) radius 1.5
  circle A5 centre (0, 59) radius 1.5
  circle A6 centre (-1, -59) radius 1.5
  point P0 (146.75, -65)
  constraint horizontal L2
  constraint vertical L3
  constraint horizontal L4
  constraint vertical L5
  constraint coincident L0.start A1.centre
  constraint coincident P0 L3.end
extrude "Extrude14" add sketch "Sketch18" along normal blind 3.5 separate body makes body 25
sketch "top" plane through (0, -55, 0) normal (0, -1, 0) x (1, 0, 0)
  circle A0 centre (140.75, 59) radius 1.5
  circle A1 centre (-140.75, -59) radius 1.5
  circle A2 centre (-140.75, 59) radius 1.5
  circle A3 centre (140.75, -59) radius 1.5
  line L0 (-146.75, -65) -> (146.75, -65)
  line L1 (146.75, -65) -> (146.75, 65)
  line L2 (146.75, 65) -> (-146.75, 65)
  line L3 (-146.75, 65) -> (-146.75, -65)
  circle A4 centre (-1, -59) radius 1.5
  circle A5 centre (0, 59) radius 1.5
sketch "middle" plane through (1.75, 0, 0) normal (1, 0, 0) x (0, 0, -1)
  line L0 (-65, -35.5) -> (-61, -35.5)
  line L1 (-61, -35.5) -> (-61, -4)
  line L2 (-61, -4) -> (61, -4)
  line L3 (61, -4) -> (61, -35.5)
  line L4 (61, -35.5) -> (65, -35.5)
  line L5 (65, -35.5) -> (65, -25.25)
  line L6 (65, -25.25) -> (68.5, -25.25)
  line L7 (68.5, -25.25) -> (68.5, -10.25)
  line L8 (68.5, -10.25) -> (65, -10.25)
  line L9 (65, -10.25) -> (65, 0)
  line L10 (65, 0) -> (12.5, 0)
  line L11 (12.5, 0) -> (12.5, 3.5)
  line L12 (12.5, 3.5) -> (-12.5, 3.5)
  line L13 (-12.5, 3.5) -> (-12.5, 0)
  line L14 (-12.5, 0) -> (-65, 0)
  line L15 (-65, 0) -> (-65, -10.25)
  line L16 (-65, -10.25) -> (-68.5, -10.25)
  line L17 (-68.5, -10.25) -> (-68.5, -25.25)
  line L18 (-68.5, -25.25) -> (-65, -25.25)
  line L19 (-65, -25.25) -> (-65, -35.5)
sketch "corner1" plane through (0, -41, 0) normal (0, 1, 0) x (-1, 0, 0)
  circle A0 centre (140.75, -59) radius 1.5
  line L0 (131.75, -65) -> (146.75, -65)
  line L1 (146.75, -65) -> (146.75, -50)
  arc A1 (146.75, -50) -> (131.75, -65) centre (146.75, -65) ccw
sketch "corner2" plane through (0, -44.5, 0) normal (0, 1, 0) x (-1, 0, 0)
  line L0 (142.5, -55.9689) -> (144.25, -59)
  line L1 (144.25, -59) -> (142.5, -62.0311)
  line L2 (142.5, -62.0311) -> (139, -62.0311)
  line L3 (139, -62.0311) -> (137.25, -59)
  line L4 (137.25, -59) -> (139, -55.9689)
  line L5 (139, -55.9689) -> (142.5, -55.9689)
  arc A0 (146.75, -50) -> (131.75, -65) centre (146.75, -65) ccw
  line L6 (131.75, -65) -> (135.25, -65)
  line L7 (135.25, -65) -> (135.25, -68.5)
  line L8 (135.25, -68.5) -> (143.25, -68.5)
  line L9 (143.25, -68.5) -> (143.25, -65)
  line L10 (143.25, -65) -> (146.75, -65)
  line L11 (146.75, -65) -> (146.75, -61.5)
  line L12 (146.75, -61.5) -> (150.25, -61.5)
  line L13 (150.25, -61.5) -> (150.25, -53.5)
  line L14 (150.25, -53.5) -> (146.75, -53.5)
  line L15 (146.75, -53.5) -> (146.75, -50)
sketch "corner3" plane through (0, -48, 0) normal (0, 1, 0) x (-1, 0, 0)
  circle A0 centre (140.75, -59) radius 1.5
  line L0 (131.75, -65) -> (146.75, -65)
  line L1 (146.75, -65) -> (146.75, -50)
  arc A1 (146.75, -50) -> (131.75, -65) centre (146.75, -65) ccw
combine "Combine10" operation cut target body 3 tool bodies 22 23 24 keep tools
combine "Combine11" operation cut target body 2 tool bodies 19 20 21 keep tools
sketch "left" plane through (0, 0, -68.5) normal (0, 0, -1) x (-1, 0, 0)
  line L0 (-9, -48) -> (-9, -44.5)
  line L1 (-9, -44.5) -> (11, -44.5)
  line L2 (11, -44.5) -> (11, -48)
  line L3 (11, -48) -> (-9, -48)
  line L4 (1.75, -25.25) -> (-1.75, -25.25)
  line L5 (-1.75, -25.25) -> (-1.75, -10.25)
  line L6 (-1.75, -10.25) -> (1.75, -10.25)
  line L7 (1.75, -10.25) -> (1.75, -25.25)
  line L8 (-143.25, -48) -> (-143.25, -44.5)
  line L9 (-143.25, -44.5) -> (-135.25, -44.5)
  line L10 (-135.25, -44.5) -> (-135.25, -48)
  line L11 (-135.25, -48) -> (-143.25, -48)
  line L12 (135.25, -48) -> (135.25, -44.5)
  line L13 (135.25, -44.5) -> (143.25, -44.5)
  line L14 (143.25, -44.5) -> (143.25, -48)
  line L15 (143.25, -48) -> (135.25, -48)
  line L16 (-150.25, -16) -> (-150.25, -35.5)
  line L17 (-150.25, -35.5) -> (-146.75, -35.5)
  line L18 (-146.75, -35.5) -> (-146.75, -55)
  line L19 (-146.75, -55) -> (146.75, -55)
  line L20 (146.75, -55) -> (146.75, -35.5)
  line L21 (146.75, -35.5) -> (150.25, -35.5)
  line L22 (150.25, -35.5) -> (150.25, -16)
  line L23 (150.25, -16) -> (146.75, -16)
  line L24 (146.75, -16) -> (146.75, 3.5)
  line L25 (146.75, 3.5) -> (107.3214, 3.5)
  line L26 (107.3214, 3.5) -> (107.3214, 0)
  line L27 (107.3214, 0) -> (64.3929, 0)
  line L28 (64.3929, 0) -> (64.3929, 3.5)
  line L29 (64.3929, 3.5) -> (21.4643, 3.5)
  line L30 (21.4643, 3.5) -> (21.4643, 0)
  line L31 (21.4643, 0) -> (-21.4643, 0)
  line L32 (-21.4643, 0) -> (-21.4643, 3.5)
  line L33 (-21.4643, 3.5) -> (-64.3929, 3.5)
  line L34 (-64.3929, 3.5) -> (-64.3929, 0)
  line L35 (-64.3929, 0) -> (-107.3214, 0)
  line L36 (-107.3214, 0) -> (-107.3214, 3.5)
  line L37 (-107.3214, 3.5) -> (-146.75, 3.5)
  line L38 (-146.75, 3.5) -> (-146.75, -16)
  line L39 (-146.75, -16) -> (-150.25, -16)
sketch "right" plane through (0, 0, 68.5) normal (0, 0, 1) x (1, 0, 0)
  line L0 (-10, -48) -> (-10, -44.5)
  line L1 (-10, -44.5) -> (10, -44.5)
  line L2 (10, -44.5) -> (10, -48)
  line L3 (10, -48) -> (-10, -48)
  line L4 (-1.75, -10.25) -> (1.75, -10.25)
  line L5 (1.75, -10.25) -> (1.75, -25.25)
  line L6 (1.75, -25.25) -> (-1.75, -25.25)
  line L7 (-1.75, -25.25) -> (-1.75, -10.25)
  line L8 (135.25, -48) -> (135.25, -44.5)
  line L9 (135.25, -44.5) -> (143.25, -44.5)
  line L10 (143.25, -44.5) -> (143.25, -48)
  line L11 (143.25, -48) -> (135.25, -48)
  line L12 (-143.25, -48) -> (-143.25, -44.5)
  line L13 (-143.25, -44.5) -> (-135.25, -44.5)
  line L14 (-135.25, -44.5) -> (-135.25, -48)
  line L15 (-135.25, -48) -> (-143.25, -48)
  line L16 (150.25, -35.5) -> (150.25, -16)
  line L17 (150.25, -16) -> (146.75, -16)
  line L18 (146.75, -16) -> (146.75, 3.5)
  line L19 (146.75, 3.5) -> (107.3214, 3.5)
  line L20 (107.3214, 3.5) -> (107.3214, 0)
  line L21 (107.3214, 0) -> (64.3929, 0)
  line L22 (64.3929, 0) -> (64.3929, 3.5)
  line L23 (64.3929, 3.5) -> (21.4643, 3.5)
  line L24 (21.4643, 3.5) -> (21.4643, 0)
  line L25 (21.4643, 0) -> (-21.4643, 0)
  line L26 (-21.4643, 0) -> (-21.4643, 3.5)
  line L27 (-21.4643, 3.5) -> (-64.3929, 3.5)
  line L28 (-64.3929, 3.5) -> (-64.3929, 0)
  line L29 (-64.3929, 0) -> (-107.3214, 0)
  line L30 (-107.3214, 0) -> (-107.3214, 3.5)
  line L31 (-107.3214, 3.5) -> (-146.75, 3.5)
  line L32 (-146.75, 3.5) -> (-146.75, -16)
  line L33 (-146.75, -16) -> (-150.25, -16)
  line L34 (-150.25, -16) -> (-150.25, -35.5)
  line L35 (-150.25, -35.5) -> (-146.75, -35.5)
  line L36 (-146.75, -35.5) -> (-146.75, -55)
  line L37 (-146.75, -55) -> (146.75, -55)
  line L38 (146.75, -55) -> (146.75, -35.5)
  line L39 (146.75, -35.5) -> (150.25, -35.5)
sketch "cornerm1" plane through (0, -51.5, 0) normal (0, -1, 0) x (1, 0, 0)
  circle A0 centre (0, 59) radius 1.5
  arc A1 (-15, 65) -> (15, 65) centre (0, 65) ccw
  line L0 (15, 65) -> (-15, 65)
sketch "cornerm2" plane through (0, -48, 0) normal (0, -1, 0) x (1, 0, 0)
  line L0 (1.75, 55.9689) -> (-1.75, 55.9689)
  line L1 (-1.75, 55.9689) -> (-3.5, 59)
  line L2 (-3.5, 59) -> (-1.75, 62.0311)
  line L3 (-1.75, 62.0311) -> (1.75, 62.0311)
  line L4 (1.75, 62.0311) -> (3.5, 59)
  line L5 (3.5, 59) -> (1.75, 55.9689)
  line L6 (-10, 65) -> (-15, 65)
  arc A0 (-15, 65) -> (15, 65) centre (0, 65) ccw
  line L7 (15, 65) -> (10, 65)
  line L8 (10, 65) -> (10, 68.5)
  line L9 (10, 68.5) -> (-10, 68.5)
  line L10 (-10, 68.5) -> (-10, 65)
sketch "cornerm3" plane through (0, -44.5, 0) normal (0, -1, 0) x (1, 0, 0)
  circle A0 centre (0, 59) radius 1.5
  arc A1 (-15, 65) -> (15, 65) centre (0, 65) ccw
  line L0 (15, 65) -> (-15, 65)
hidden bodies 6 7
equation "d7 = boardT"
equation "boardT = 3.5 mm"
equation "d9 = boardT"
equation "d10 = boardT"
equation "d11 = boardT"
equation "d12 = boardT"
equation "d18 = -boardT"
equation "d22 = boardT"
equation "d23 = boardT"
equation "d24 = boardT"
equation "d26 = -boardT"
equation "d28 = -boardT"
equation "d31 = boardT"
equation "d32 = -boardT"
equation "d34 = -boardT"
equation "d54 = -boardT"
equation "d57 = -boardT"
equation "d59 = -3 * boardT"
equation "d61 = -boardT"
equation "d62 = -boardT"
equation "d64 = boardT"
equation "d67 = boardT"
equation "d72 = -boardT"
equation "d75 = -3 * boardT"
equation "d78 = boardT"
equation "d86 = boardT"
equation "d89 = boardT"
equation "d91 = boardT"
equation "d94 = boardT"
equation "d96 = -boardT"
equation "d99 = -boardT"
equation "d102 = boardT"
equation "d105 = boardT"
equation "d108 = boardT"
